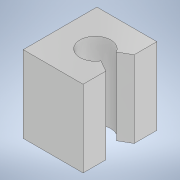
# Autodesk Inventor part: Rodamiento lineal
Saved by Autodesk Inventor 2021 (Build 250183000, 183)
## iProperties
Created: 2022-02-08
Part Number: Rodamiento lineal
Material: Generic
Document SubType Name: Modeling
Designer: deuts
Density: 1 g/cm^3
Appearance: Default
Author: deuts
Autodesk Inventor part; units mm, degrees
ref_plane "YZ Plane" through (0, 0, 0) normal (1, 0, 0) x (0, 1, 0)
ref_plane "XZ Plane" through (0, 0, 0) normal (0, 1, 0) x (-1, 0, 0)
ref_plane "XY Plane" through (0, 0, 0) normal (0, 0, 1) x (1, 0, 0)
sketch "Sketch1" plane through (0, 0, 0) normal (0, 1, 0) x (-1, 0, 0)
  arc A0 (-8.6603, -5) -> (-8.6603, 5) centre (0, 0) ccw
  line L0 (-8.6603, -5) -> (-16, -9.2376)
  line L1 (-8.6603, 5) -> (-16, 9.2376)
  line L2 (0, 0) -> (23, 0)
  line L3 (23, 0) -> (23, -24)
  line L4 (23, 0) -> (23, 24)
  line L5 (23, -24) -> (-16, -24)
  line L6 (-16, -24) -> (-16, -9.2376)
  line L7 (23, 24) -> (-16, 24)
  line L8 (-16, 24) -> (-16, 9.2376)
  dimension "d0" = 20
  dimension "d2" = 23
  dimension "d3" = 24
  dimension "d4" = 24
  dimension "d5" = 39
  constraints: 18 end point, 3 point on line, 2 horizontal, 2 perpendicular, 2 point on circle, 1 centre point, 1 coincident, 1 vertical
  measures "d0" diameter of A0
  measures "d2" distance of L2.start L2.end
  measures "d3" distance of L2.end L3.end
  measures "d4" distance of L2.end L4.end
  measures "d5" distance of L3.end L5.end
extrude "Extrusion1" add sketch "Sketch1" along normal blind 50
sketch "Sketch2" plane through (-23, 0, -24) normal (-1, 0, 0) x (0, 0, 1)
  line L0 (48, 0) -> (48, 50) projected
  line L1 (14.7624, 0) -> (0, 0) projected
  line L2 (48, 0) -> (33.2376, 0) projected
  line L3 (14.7624, 50) -> (0, 50) projected
  circle A0 centre (6.5, 42.5) radius 3
  circle A1 centre (6.5, 7.5) radius 3
  circle A2 centre (41.5, 7.5) radius 3
  circle A3 centre (41.5, 42.5) radius 3
  point P0 (24, 0)
  point P1 (24, 25)
  dimension "d10" = 6
  dimension "d11" = 6
  dimension "d12" = 6
  dimension "d13" = 6
  constraints: 4 centre point
  measures "d10" diameter of A0
  measures "d11" diameter of A1
  measures "d12" diameter of A2
  measures "d13" diameter of A3
extrude "Extrusion2" cut sketch "Sketch2" against normal blind 12
body "Solid1"
